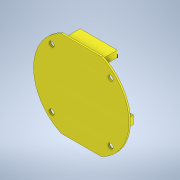
# Autodesk Inventor part: Zestaw startowy Cansat
Saved by Autodesk Inventor 2020 (Build 240168000, 168)
## iProperties
Created: 2021-10-10
Part Number: Zestaw startowy Cansat
Material: Ogólny
Document SubType Name: Modeling
Designer: Komputer
Density: 1 g/cm^3
Appearance: Kanarkowa
Author: Komputer
Autodesk Inventor part; units mm, degrees
ref_plane "YZ Plane" through (0, 0, 0) normal (1, 0, 0) x (0, 1, 0)
ref_plane "XZ Plane" through (0, 0, 0) normal (0, 1, 0) x (-1, 0, 0)
ref_plane "XY Plane" through (0, 0, 0) normal (0, 0, 1) x (1, 0, 0)
sketch "Szkic1" plane through (0, 0, 0) normal (0, 0, 1) x (1, 0, 0)
  circle A0 centre (0, 0) radius 30
  line L0 (0, 0) -> (0, 27.2)
  line L1 (0, 0) -> (0, -27.2)
  line L2 (0, -27.2) -> (12.6554, -27.2)
  line L3 (0, -27.2) -> (-12.6554, -27.2)
  line L4 (0, 27.2) -> (12.6554, 27.2)
  line L5 (0, 27.2) -> (-12.6554, 27.2)
  line L6 (0, 0) -> (0, 18.5)
  line L7 (0, 18.5) -> (-18.5, 18.5)
  line L8 (0, 18.5) -> (18.5, 18.5)
  line L9 (18.5, 18.5) -> (18.5, -18.5)
  line L10 (18.5, -18.5) -> (-18.5, -18.5)
  circle A1 centre (18.5, 18.5) radius 1.6
  circle A2 centre (18.5, -18.5) radius 1.6
  circle A3 centre (-18.5, -18.5) radius 1.6
  circle A4 centre (-18.5, 18.5) radius 1.6
  dimension "d0" = 60
  dimension "d1" = 27.2
  dimension "d2" = 27.2
  dimension "d3" = 18.5
  dimension "d4" = 18.5
  dimension "d5" = 18.5
  dimension "d6" = 37
  dimension "d7" = 37
  dimension "d8" = 3.2
  dimension "d9" = 3.2
  dimension "d10" = 3.2
  dimension "d11" = 3.2
  constraints: 22 end point, 5 centre point, 5 coincident, 4 perpendicular, 4 point on circle, 3 point on line, 2 vertical, 1 horizontal, 1 parallel
  measures "d0" diameter of A0
  measures "d1" distance of L0.start L0.end
  measures "d2" distance of L0.start L1.end
  measures "d3" distance of L0.start L6.end
  measures "d4" distance of L6.end L7.end
  measures "d5" distance of L6.end L8.end
  measures "d6" distance of L8.end L9.end
  measures "d7" distance of L9.end L10.end
  measures "d8" diameter of A1
  measures "d9" diameter of A2
  measures "d10" diameter of A3
  measures "d11" diameter of A4
extrude "Wyciągnięcie proste1" add sketch "Szkic1" along normal blind 1 contours A0 L2 L1 L10 A2 L9 A1 L8 L0 L4 | L5 L0 L1 L3 A0 | L8 A1 L9 A2 L10 L1 L0
sketch "Szkic2" plane through (0, 0, 0) normal (0, 0, -1) x (-1, 0, 0)
  line L0 (0, 0) -> (0, -21.6)
  line L1 (0, -21.6) -> (8.8, -21.6)
  line L2 (8.8, -21.6) -> (8.8, -24)
  line L3 (8.8, -24) -> (-8.8, -24)
  line L4 (-8.8, -24) -> (-8.8, -21.6)
  line L5 (-8.8, -21.6) -> (0, -21.6)
  line L6 (9.5, -25) -> (-9.5, -25)
  line L7 (-9.5, -25) -> (-9.5, -21)
  line L8 (-9.5, -21) -> (9.5, -21)
  line L9 (9.5, -21) -> (9.5, -25)
  line L10 (9.5, -25) -> (-9.5, -21) construction
  line L11 (-9.5, -25) -> (9.5, -21) construction
  line L12 (0, 0) -> (0, 22.8)
  line L13 (11.7, 20.8) -> (-11.7, 20.8)
  line L14 (-11.7, 20.8) -> (-11.7, 24.8)
  line L15 (-11.7, 24.8) -> (11.7, 24.8)
  line L16 (11.7, 24.8) -> (11.7, 20.8)
  line L17 (11.7, 20.8) -> (-11.7, 24.8) construction
  line L18 (-11.7, 20.8) -> (11.7, 24.8) construction
  arc A0 (-12.6554, 27.2) -> (-12.6554, -27.2) centre (0, 0) ccw projected
  line L19 (-25.1113, -2.5816) -> (-29.8887, -2.5816)
  line L20 (-29.8887, -2.5816) -> (-29.8887, 2.5816)
  line L21 (-29.8887, 2.5816) -> (-25.1113, 2.5816)
  line L22 (-25.1113, 2.5816) -> (-25.1113, -2.5816)
  line L23 (-25.1113, -2.5816) -> (-29.8887, 2.5816) construction
  line L24 (-29.8887, -2.5816) -> (-25.1113, 2.5816) construction
  line L25 (12.5, -7.5) -> (27.5, -7.5)
  line L26 (27.5, -7.5) -> (27.5, 7.5)
  line L27 (27.5, 7.5) -> (12.5, 7.5)
  line L28 (12.5, 7.5) -> (12.5, -7.5)
  line L29 (12.5, -7.5) -> (27.5, 7.5) construction
  line L30 (27.5, -7.5) -> (12.5, 7.5) construction
  point P0 (0, -23)
  point P1 (-27.5, 0)
  point P2 (20, 0)
  dimension "d14" = 21.6
  dimension "d15" = 8.8
  dimension "d16" = 2.4
  dimension "d17" = 17.6
  dimension "d19" = 19
  dimension "d20" = 4
  dimension "d21" = 22.8
  dimension "d22" = 23.4
  dimension "d23" = 4
  dimension "d24" = 15
  dimension "d25" = 15
  constraints: 62 end point, 9 perpendicular, 8 midpoint, 8 parallel, 4 horizontal, 2 vertical, 1 point on circle, 1 point on line
  measures "d14" distance of L0.start L0.end
  measures "d15" distance of L0.end L1.end
  measures "d16" distance of L1.end L2.end
  measures "d17" distance of L2.end L3.end
  measures "d19" distance of L7.end L8.end
  measures "d20" distance of L6.end L7.end
  measures "d21" distance of L0.start L12.end
  measures "d22" distance of L14.end L15.end
  measures "d23" distance of L13.end L14.end
  measures "d24" distance of L27.end L26.end
  measures "d25" distance of L26.end L25.end
extrude "Wyciągnięcie proste2" add sketch "Szkic2" along normal blind 2 contours L1 L2 L3 L4 L5 | L6 L7 L8 L9 | L13 L14 L15 L16 | L21 L22 L19 L20 | L28 L27 L26 L25
sketch "Szkic3" plane through (0, 0, -2) normal (0, 0, -1) x (-1, 0, 0)
  line L0 (-9.5, -21) -> (-9.5, -25) projected
  line L1 (-9.5, -21) -> (9.5, -21) projected
  line L2 (-9.5, -21) -> (9.5, -21)
  line L3 (9.5, -21) -> (9.5, -25) projected
  line L4 (9.5, -21) -> (9.5, -25)
  line L5 (-9.5, -25) -> (9.5, -25) projected
  line L6 (9.5, -25) -> (-9.5, -25)
  line L7 (-9.5, -25) -> (-9.5, -21)
  line L8 (11.7, 24.8) -> (-11.7, 24.8) projected
  line L9 (-11.7, 24.8) -> (11.7, 24.8)
  line L10 (11.7, 20.8) -> (11.7, 24.8) projected
  line L11 (11.7, 24.8) -> (11.7, 20.8)
  line L12 (-11.7, 20.8) -> (11.7, 20.8) projected
  line L13 (11.7, 20.8) -> (-11.7, 20.8)
  line L14 (-11.7, 20.8) -> (-11.7, 24.8) projected
  line L15 (-11.7, 20.8) -> (-11.7, 24.8)
  point P0 (0, 0)
  constraints: 16 end point, 4 collinear, 3 perpendicular, 1 horizontal
extrude "Wyciągnięcie proste3" add sketch "Szkic3" along normal blind 8
sketch "Szkic4" plane through (0, 0, -10) normal (0, 0, -1) x (-1, 0, 0)
  line L0 (-11.7, 20.8) -> (-11.7, 24.8) projected
  line L1 (-11.7, 20.8) -> (-11.7, 22.8)
  line L2 (-11.7, 22.8) -> (11.7, 22.8)
  line L3 (11.7, 24.8) -> (11.7, 20.8) projected
  point P0 (0, 0)
  constraints: 4 end point, 2 midpoint
sketch "Szkic5" plane through (0, 0, 0) normal (0, 0, -1) x (-1, 0, 0)
  point P0 (0, 0)
